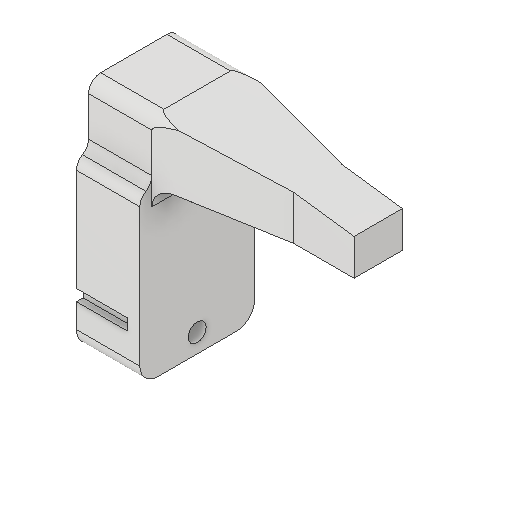
# Autodesk Inventor part: 3DP_PLA_X_axis_carriage_belt_mount
Saved by Autodesk Inventor 2026.1 (Build 301233000, 233)
## iProperties
Created: 2018-07-07
Part Number: 3DP_PLA_X_axis_carriage_belt_mount
Material: ABS Plastic
Document SubType Name: Modeling
Designer: Andrzej
Density: 1.06 g/cm^3
Appearance: Smooth - White
Author: Andrzej
Autodesk Inventor part; units mm, degrees
ref_plane "YZ Plane" through (0, 0, 0) normal (1, 0, 0) x (0, 1, 0)
ref_plane "XZ Plane" through (0, 0, 0) normal (0, 1, 0) x (-1, 0, 0)
ref_plane "XY Plane" through (0, 0, 0) normal (0, 0, 1) x (1, 0, 0)
sketch "Sketch1" plane through (0, 0, 0) normal (1, 0, 0) x (0, 1, 0)
  line L0 (16.8586, 5.2751) -> (-11.0014, 5.2751)
  line L1 (-11.0014, 5.2751) -> (-11.0014, -13.7249)
  line L2 (-11.0014, -13.7249) -> (16.8586, -13.7249)
  line L3 (16.8586, -13.7249) -> (16.8586, 5.2751)
  line L4 (-2.1014, 5.2751) -> (-2.1014, -13.7249)
  line L5 (-4.0014, 5.2751) -> (-4.0014, -13.7249)
  point P0 (0, 0)
  point P1 (12.3586, -4.2249)
  point P2 (-7.8914, -4.2249)
  dimension "d1" = 19
  dimension "d2" = 1.9
  dimension "d3" = 18.96
  dimension "d4" = 7
  dimension "d19" = 9.5
  dimension "d39" = 20.25
  dimension "d40" = 4.5
  constraints: 12 end point, 4 point on line, 3 perpendicular, 2 parallel, 1 horizontal, 1 horizontal alignment
  measures "d1" distance of L1.end L0.end
  measures "d2" distance between parallel lines of L5 L4
  measures "d3" distance between parallel lines of L3 L4
  measures "d4" distance between parallel lines of L1 L5
  measures "d19" distance from line of L2 point (12.359, -4.225)
  measures "d39" distance of point (12.359, -4.225) point (-7.891, -4.225)
  measures "d40" distance from line of L3 point (12.359, -4.225)
extrude "Extrusion1" add sketch "Sketch1" along normal blind 8.5 contours L3 L2 L4 L0 | L5 L2 L1 L0
sketch "Sketch2" plane through (8.5, 0, 0) normal (1, 0, 0) x (0, 0, -1)
  line L0 (-5.2751, 16.8586) -> (-5.2751, -2.1014) projected
  line L1 (-5.2751, -2.1014) -> (13.7249, -2.1014) projected
  line L2 (13.7249, -2.1014) -> (13.7249, 16.8586) projected
  line L3 (13.7249, 16.8586) -> (-5.2751, 16.8586) projected
  line L4 (13.7249, -11.0014) -> (13.7249, -4.0014) projected
  line L5 (13.7249, -4.0014) -> (-5.2751, -4.0014) projected
  line L6 (-5.2751, -4.0014) -> (-5.2751, -11.0014) projected
  line L7 (-5.2751, -11.0014) -> (13.7249, -11.0014) projected
  line L8 (-5.2751, -2.1014) -> (-5.2751, -4.0014)
  line L9 (13.7249, -2.1014) -> (13.7249, 16.8586) projected
  line L10 (13.7249, -11.0014) -> (13.7249, -4.0014) projected
  line L11 (13.7249, -2.1014) -> (13.7249, -4.0014)
  point P0 (0, 0)
  constraints: 4 end point, 2 vertical
extrude "Extrusion2" add sketch "Sketch2" along normal blind 2
sketch "Sketch3" plane through (0, 0, 0) normal (-1, 0, 0) x (0, 0, 1)
  line L0 (-13.7249, -11.0014) -> (-13.7249, -4.0014) projected
  line L1 (5.2751, -11.0014) -> (-13.7249, -11.0014) projected
  line L2 (5.2751, -4.0014) -> (5.2751, -11.0014) projected
  line L3 (-13.7249, -4.0014) -> (5.2751, -4.0014) projected
  line L4 (5.2751, 16.8586) -> (5.2751, -2.1014) projected
  line L5 (-13.7249, 16.8586) -> (5.2751, 16.8586) projected
  line L6 (-13.7249, -2.1014) -> (-13.7249, 16.8586) projected
  line L7 (5.2751, -2.1014) -> (-13.7249, -2.1014) projected
  line L8 (-12.6249, -4.0014) -> (-11.8249, -4.0014)
  line L9 (-11.8249, -4.0014) -> (-11.8249, -3.0014)
  line L10 (-11.8249, -3.0014) -> (-12.6249, -3.0014)
  line L11 (-12.6249, -3.0014) -> (-12.6249, -4.0014)
  point P0 (0, 0)
  dimension "d9" = 1
  dimension "d10" = 0.8
  dimension "d11" = 1.1
  constraints: 8 end point, 2 parallel, 1 horizontal, 1 perpendicular, 1 point on line
  measures "d9" distance between parallel lines of L3 L10
  measures "d10" distance between parallel lines of L11 L9
  measures "d11" distance between parallel lines of L0 L11
extrude "Extrusion3" add sketch "Sketch3" against normal up to surface (8.5 mm away) contours L11 L10 L9 L3
fillet "Fillet1" radius 0.2 2 edges at (4.25, -3.0014, -12.6249) (4.25, -3.0014, -11.8249)
pattern_linear "Rectangular Pattern1" count 9 spacing 2 along (0, 0, 1) of "Extrusion3", "Fillet1"
hole "Hole2" at (0, 12.3586, -4.2249) at (0, -7.8914, -4.2249) direction (1, 0, 0) diameter 3 end through all
fillet "Fillet3" radius 3 2 edges at (5.25, -11.0014, -13.7249) (5.25, -11.0014, 5.2751)
fillet "Fillet3" radius 2 2 edges at (5.25, 16.8586, 5.2751) (5.25, 16.8586, -13.7249)
sketch "Sketch4" plane through (0, 16.8586, 3.2751) normal (0, 1, 0) x (1, 0, 0)
  line L0 (0, 15) -> (10.5, 15) projected
  line L1 (0, 15) -> (0, 0) projected
  line L2 (10.5, 0) -> (0, 0) projected
  line L3 (10.5, 15) -> (10.5, 0) projected
  line L4 (10.5, 17) -> (10.5, 15) projected
  line L5 (10.5, 15) -> (30.5, 15)
  line L6 (30.5, 15) -> (30.5, 0)
  line L7 (30.5, 0) -> (10.5, 0)
  line L8 (30.5, 11.5) -> (40.5, 11.5)
  line L9 (40.5, 11.5) -> (40.5, 3.5)
  line L10 (40.5, 3.5) -> (30.5, 3.5)
  point P0 (0, 3.2751)
  dimension "d50" = 20
  dimension "d51" = 15
  dimension "d52" = 8
  dimension "d53" = 3.5
  dimension "d54" = 10
  constraints: 12 end point, 3 perpendicular, 2 horizontal, 2 point on line, 1 collinear
  measures "d50" distance between parallel lines of L3 L6
  measures "d51" distance of L0.start L1.end
  measures "d52" distance of L8.end L9.end
  measures "d53" distance between parallel lines of L5 L8
  measures "d54" distance of L8.start L8.end
extrude "Extrusion4" add sketch "Sketch4" along normal blind 10
chamfer "Chamfer4" distance 20 distance2 3.5 1 edges at (30.5, 21.8586, 3.2751) measured on face at (13.6667, 23.5253, 3.2751)
chamfer "Chamfer5" distance 20 distance2 3.5 1 edges at (30.5, 21.8586, -11.7249) measured on face at (13.6667, 23.5253, -11.7249)
chamfer "Chamfer6" distance 30 distance2 4 1 edges at (40.5, 26.8586, -4.2249) measured on face at (17.167, 26.8586, -2.8915)
fillet "Fillet4" radius 2 4 edges at (5.25, 16.8586, 3.2751) (5.25, 26.8586, 3.2751) (5.25, 26.8586, -11.7249) (5.25, 16.8586, -11.7249)
fillet "Fillet4" radius 3 1 edges at (10.5, 16.8586, -4.2249)
sketch "Sketch5" plane through (10.5, -8.0014, 5.2751) normal (1, 0, 0) x (0, 0, -1)
  line L0 (2, 26.3241) -> (2, 21.86) projected
  arc A0 (1, 24.5921) -> (2, 26.3241) centre (0, 26.3241) ccw projected
  arc A1 (1, 24.5921) -> (0, 22.86) centre (2, 22.86) ccw projected
  line L1 (0, 22.86) -> (0, 0) projected
  arc A2 (0, 0) -> (3, -3) centre (3, 0) ccw projected
  line L2 (3, -3) -> (16, -3) projected
  arc A3 (16, -3) -> (19, 0) centre (16, 0) ccw projected
  line L3 (19, 0) -> (19, 22.86) projected
  arc A4 (19, 22.86) -> (18, 24.5921) centre (17, 22.86) ccw projected
  arc A5 (17, 26.3241) -> (18, 24.5921) centre (19, 26.3241) ccw projected
  line L4 (17, 21.86) -> (17, 26.3241) projected
  line L5 (9.5, 21.86) -> (17, 21.86) projected
  circle A6 centre (9.5, 20.36) radius 1.5 projected
  line L6 (2, 21.86) -> (9.5, 21.86) projected
  circle A7 centre (9.5, 0.11) radius 1.5 projected
  circle A8 centre (9.5, 20.36) radius 1.5 projected
  circle A9 centre (9.5, 20.36) radius 3
  point P0 (5.2751, 8.0014)
  dimension "d68" = 6
  constraints: 2 vertical alignment, 1 centre point, 1 coincident
  measures "d68" diameter of A9
extrude "Extrusion5" cut sketch "Sketch5" along normal blind 10 contours A9 L5 L6 | L6 L5 A9
sketch "Sketch6" plane through (30.5, 16.8586, -0.2249) normal (0, 0, 1) x (1, 0, 0)
  point P0 (-30.5, -16.8586)
equation "\"d19\" = 0.5 * d1"
equation "\"d53\" = -0.5 * d52 + 0.5 * d51"
body "Solid1"
